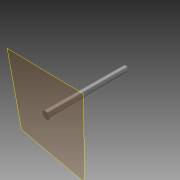
# Autodesk Inventor part: stepperMotorAxel
Saved by Autodesk Inventor 2013 (Build 170138000, 138)
## iProperties
Created: 2013-02-24
Part Number: stepperMotorAxel
Material: Steel, Alloy
Document SubType Name: Modeling
Designer: Nano
Mass: 16.4061 g
Surface Area: 14.1427 cm^2
Volume: 2.08995 cm^3
Density: 7.85 g/cm^3
Author: Nano
Autodesk Inventor part; units mm, degrees
ref_plane "YZ Plane" through (0, 0, 0) normal (1, 0, 0) x (0, 1, 0)
ref_plane "XZ Plane" through (0, 0, 0) normal (0, 1, 0) x (-1, 0, 0)
ref_plane "XY Plane" through (0, 0, 0) normal (0, 0, 1) x (1, 0, 0)
ref_plane "Work Plane1" through (0, 0, 0) normal (0, 0, 1) x (1, 0, 0)
sketch "Sketch1" plane through (0, 0, 0) normal (0, 0, 1) x (1, 0, 0)
  circle A0 centre (0, 0) radius 3.0861
  point P0 (0, 0)
  dimension "d2" = 6.1722
  constraints: 1 centre point
  measures "d2" diameter of A0
extrude "Extrusion1" add sketch "Sketch1" against normal blind 69.85
body "Solid1"
